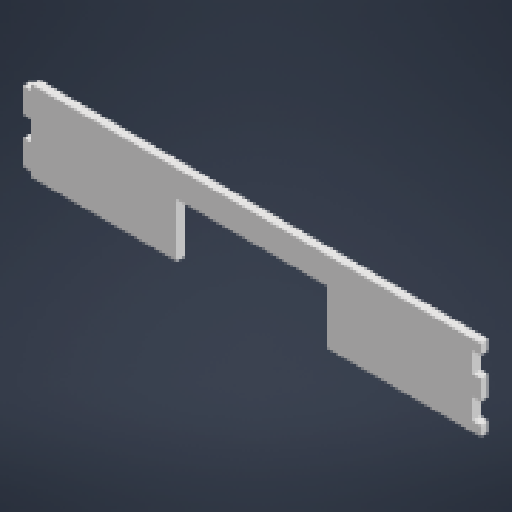
# Autodesk Inventor part: Pieza1
Saved by Autodesk Inventor 2026.1 (Build 301233020, 233B)
## iProperties
Created: 2026-05-06
Part Number: Pieza1
Material: Genérico
Document SubType Name: Modeling
Designer: OlmesTech
Density: 1 g/cm^3
Appearance: Valor por defecto
Author: OlmesTech
Autodesk Inventor part; units mm, degrees
ref_plane "YZ Plane" through (0, 0, 0) normal (1, 0, 0) x (0, 1, 0)
ref_plane "XZ Plane" through (0, 0, 0) normal (0, 1, 0) x (-1, 0, 0)
ref_plane "XY Plane" through (0, 0, 0) normal (0, 0, 1) x (1, 0, 0)
sketch "Boceto1" plane through (0, 0, 0) normal (0, 0, 1) x (1, 0, 0)
  line L0 (85, 15) -> (-82, 15)
  line L1 (-85, -15) -> (85, 15) construction
  line L2 (85, -15) -> (-85, 15) construction
  line L3 (-28, -15) -> (-28, 5)
  line L4 (28, 5) -> (28, -15)
  line L5 (-28, 5) -> (28, 5)
  line L6 (-82, -15) -> (-28, -15)
  line L7 (28, -15) -> (85, -15)
  line L8 (-82, -13.0321) -> (-82, -3.7)
  line L9 (-82, -3.7) -> (-85, -3.7) projected
  line L10 (-85, -13.0321) -> (-85, -3.7) projected
  line L11 (-82, -13.0321) -> (-85, -13.0321) projected
  line L12 (-82, 3.7) -> (-82, 13.0321)
  line L13 (-82, 13.0321) -> (-85, 13.0321) projected
  line L14 (-85, 3.7) -> (-85, 13.0321) projected
  line L15 (-82, 3.7) -> (-85, 3.7) projected
  line L16 (-82, -3.7) -> (-82, 3.7) projected
  line L17 (-82, 13.0321) -> (-82, 15) projected
  line L18 (-82, -15) -> (-82, -13.0321) projected
  line L19 (82, 15) -> (82, 11.3) projected
  line L20 (82, 11.3) -> (85, 11.3) projected
  line L21 (85, 15) -> (85, 11.3) projected
  line L22 (82, 15) -> (85, 15) projected
  line L23 (82, 3.7) -> (82, -3.7) projected
  line L24 (82, -3.7) -> (85, -3.7) projected
  line L25 (85, 3.7) -> (85, -3.7) projected
  line L26 (82, 3.7) -> (85, 3.7) projected
  line L27 (82, -11.3) -> (82, -15) projected
  line L28 (82, -15) -> (85, -15) projected
  line L29 (85, -11.3) -> (85, -15) projected
  line L30 (82, -11.3) -> (85, -11.3) projected
  line L31 (82, -3.7) -> (82, -11.3) projected
  line L32 (82, 11.3) -> (82, 3.7) projected
  point P0 (0, 0)
  point P1 (28, 0)
  dimension "d0" = 30
  dimension "d1" = 170
  dimension "d7" = 20
  dimension "d11" = 30
  constraints: 20 end point, 4 perpendicular, 2 horizontal, 2 midpoint, 2 parallel, 1 point on line
  measures "d0" distance of L2.start L0.start
  measures "d1" distance of L0.start L2.end
  measures "d7" distance between parallel lines of L7 L5
  measures "d11" distance of L0.end L6.start
extrude "Extrusión1" add sketch "Boceto1" along normal blind 3
